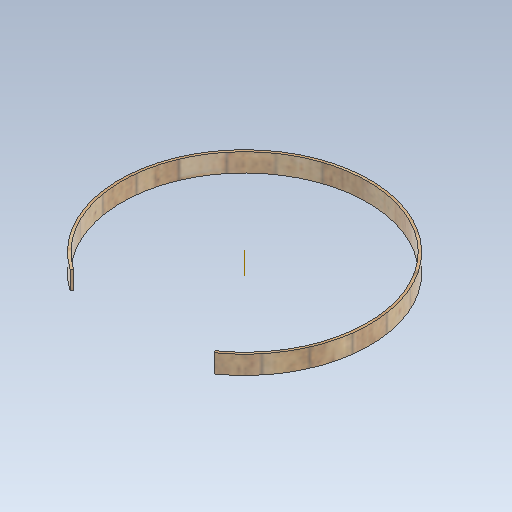
# Autodesk Inventor part: Banding Base
Saved by Autodesk Inventor 2020 (Build 240168000, 168)
## iProperties
Created: 2020-03-07
Part Number: Banding Base
Material: Wood (Maple)
Document SubType Name: Sheet Metal
Designer: Daniel Wikman
Density: 0.67 g/cm^3
Sheet Metal Rule: Default_mm
Appearance: Natural Maple - Glossy Dark Tint
Author: Daniel Wikman
Autodesk Inventor part; units mm, degrees
ref_plane "YZ Plane" through (0, 0, 0) normal (1, 0, 0) x (0, 1, 0)
ref_plane "XZ Plane" through (0, 0, 0) normal (0, 1, 0) x (-1, 0, 0)
ref_plane "XY Plane" through (0, 0, 0) normal (0, 0, 1) x (1, 0, 0)
sketch "Sketch1" plane through (0, 0, 0) normal (0, 1, 0) x (-1, 0, 0)
  arc A0 (-115.1168, 163.5486) -> (115.1168, 163.5486) centre (0, 0) ccw
  arc A1 (-117.4682, 166.785) -> (117.4682, 166.785) centre (0, 0) ccw
  line L0 (115.1168, 163.5486) -> (117.4682, 166.785)
  line L1 (-115.1168, 163.5486) -> (-117.4682, 166.785)
  dimension "d0" = 400
  dimension "d20" = 408
  constraints: 4 end point, 4 point on circle, 2 centre point, 2 coincident
  measures "d0" diameter of A0
  measures "d20" diameter of A1
extrude "Extrusion1" add sketch "Sketch1" along normal blind 30
equation "\"BendRadius\" = Thickness"
equation "\"BendReliefWidth\" = Thickness"
equation "\"BendReliefDepth\" = 0.5 * Thickness"
equation "\"CornerReliefSize\" = 4 * Thickness"
equation "\"MinimumRemnant\" = 2 * Thickness"
equation "\"TransitionRadius\" = BendRadius"
equation "\"JacobiRadiusSize\" = BendRadius"
equation "\"GapSize\" = Thickness"
equation "\"Thickness\" = 0.5"
body "Solid1"
